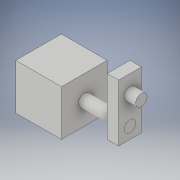
# Autodesk Inventor part: SkeletalStuff
Saved by Autodesk Inventor 2019 (Build 230136000, 136)
## iProperties
Created: 2019-04-11
Part Number: SkeletalStuff
Material: Generic
Document SubType Name: Modeling
Designer: User
Density: 1 g/cm^3
Appearance: Default
Author: User
Autodesk Inventor part; units mm, degrees
ref_plane "YZ Plane" through (0, 0, 0) normal (1, 0, 0) x (0, 1, 0)
ref_plane "XZ Plane" through (0, 0, 0) normal (0, 1, 0) x (-1, 0, 0)
ref_plane "XY Plane" through (0, 0, 0) normal (0, 0, 1) x (1, 0, 0)
sketch "Sketch1" plane through (0, 0, 0) normal (1, 0, 0) x (0, 1, 0)
  line L0 (0, 0) -> (50.8, 0)
  line L1 (50.8, 0) -> (50.8, -50.8)
  line L2 (50.8, -50.8) -> (0, -50.8)
  line L3 (0, -50.8) -> (0, 0)
  dimension "d0" = 50.8
  dimension "d1" = 50.8
  constraints: 8 end point, 2 parallel, 1 horizontal, 1 perpendicular
  measures "d0" distance of L1.end L2.end
  measures "d1" distance of L0.end L1.end
extrude "Extrusion1" add sketch "Sketch1" along normal blind 50.8
sketch "Sketch2" plane through (50.8, 0, 0) normal (1, 0, 0) x (0, 0, -1)
  circle A0 centre (25.4, 25.4) radius 6.35
  line L0 (0, 50.8) -> (0, 0) projected
  line L1 (0, 0) -> (50.8, 0) projected
  dimension "d4" = 12.7
  dimension "d5" = 25.4
  dimension "d6" = 25.4
  constraints: 1 centre point
  measures "d4" diameter of A0
  measures "d5" distance from line of L0 A0.centre
  measures "d6" distance from line of L1 A0.centre
extrude "Extrusion2" add sketch "Sketch2" along normal blind 50.8 separate body
sketch "Sketch3" plane through (101.6, 25.4, -25.4) normal (1, 0, 0) x (0, 0, -1)
  line L0 (-12.7, -12.7) -> (12.7, -12.7)
  line L1 (12.7, -12.7) -> (12.7, 50.8)
  line L2 (12.7, 50.8) -> (-12.7, 50.8)
  line L3 (-12.7, 50.8) -> (-12.7, -12.7)
  circle A0 centre (0, 0) radius 6.35 projected
  point P0 (-25.4, -25.4)
  dimension "d9" = 25.4
  dimension "d10" = 63.5
  dimension "d11" = 12.7
  dimension "d12" = 12.7
  dimension "d16" = 12.7
  constraints: 8 end point, 2 parallel, 1 horizontal, 1 perpendicular
  measures "d9" distance of L2.end L1.end
  measures "d10" distance of L1.end L0.end
  measures "d11" distance from line of L0 A0.centre
  measures "d12" diameter of A0
  measures "d16" distance from line of A0.centre L3
extrude "Extrusion3" add sketch "Sketch3" against normal blind 12.7 separate body
sketch "Sketch5" plane through (101.6, 25.4, -25.4) normal (1, 0, 0) x (0, 0, -1)
  circle A0 centre (0, 31.75) radius 6.35
  line L0 (12.7, 50.8) -> (-12.7, 50.8) projected
  line L1 (-12.7, 50.8) -> (-12.7, -12.7) projected
  point P0 (-25.4, -25.4)
  dimension "d20" = 12.7
  dimension "d21" = 25.4
  dimension "d22" = 12.7
  dimension "d23" = 19.05
  constraints: 1 centre point
  measures "d20" diameter of A0
  measures "d21" distance of L0.start L0.end
  measures "d22" distance from line of L1 A0.centre
  measures "d23" distance from line of L0 A0.centre
extrude "Extrusion6" add sketch "Sketch5" along normal blind 12.7 separate body
equation "\"d22\" = 0.5 * d21"
body "Solid1"
body "Solid2"
body "Solid3"
body "Solid6"
